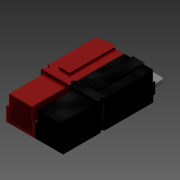
# Autodesk Inventor part: PowerPoles
Saved by Autodesk Inventor 2013 (Build 170138000, 138)
## iProperties
Created: 2012-09-17
Part Number: PowerPoles
Material: Generic
Document SubType Name: Modeling
Designer: Bail
Density: 1 g/cm^3
Author: Bail
Autodesk Inventor part; units mm, degrees
ref_plane "YZ Plane" through (0, 0, 0) normal (1, 0, 0) x (0, 1, 0)
ref_plane "XZ Plane" through (0, 0, 0) normal (0, 1, 0) x (-1, 0, 0)
ref_plane "XY Plane" through (0, 0, 0) normal (0, 0, 1) x (1, 0, 0)
sketch "Sketch1" plane through (0, 0, 0) normal (0, 0, 1) x (1, 0, 0)
  line L0 (-3.937, 3.937) -> (3.937, 3.937)
  line L1 (3.937, 3.937) -> (3.937, -3.937)
  line L2 (3.937, -3.937) -> (-3.937, -3.937)
  line L3 (-3.937, -3.937) -> (-3.937, 3.937)
  point P0 (0, 0)
  dimension "d0" = 7.874
  dimension "d2" = 7.874
  dimension "d3" = 3.937
  dimension "d4" = 3.937
  constraints: 8 end point, 2 parallel, 1 horizontal, 1 perpendicular
  measures "d0" distance of L0.start L0.end
  measures "d2" distance of L0.end L1.end
  measures "d3" distance from line of point (0, 0) L3
  measures "d4" distance from line of point (0, 0) L0
extrude "Extrusion1" add sketch "Sketch1" along normal blind 24.638
sketch "Sketch2" plane through (-3.937, 3.937, 0) normal (0, 1, 0) x (1, 0, 0)
  line L0 (0, 0) -> (7.874, 0) projected
  line L1 (0, 0) -> (0, -24.638) projected
  line L2 (7.874, 0) -> (7.874, -24.638) projected
  line L3 (2.3495, 0) -> (5.5245, 0)
  line L4 (5.5245, 0) -> (5.5245, -12.7)
  line L5 (5.5245, -12.7) -> (2.3495, -12.7)
  line L6 (2.3495, -12.7) -> (2.3495, 0)
  point P0 (3.937, 0)
  dimension "d7" = 3.175
  dimension "d9" = 2.3495
  dimension "d10" = 7.874
  dimension "d11" = 12.7
  constraints: 8 end point, 2 parallel, 1 horizontal, 1 perpendicular, 1 point on line
  measures "d7" distance of L4.end L5.end
  measures "d9" distance between parallel lines of L1 L6
  measures "d10" distance between parallel lines of L2 L1
  measures "d11" distance between parallel lines of L0 L5
extrude "Extrusion2" add sketch "Sketch2" along normal blind 0.508
sketch "Sketch3" plane through (0, 0, 0) normal (0, 0, -1) x (-1, 0, 0)
  line L0 (1.5875, 3.937) -> (1.5875, 4.445) projected
  line L1 (-1.5875, 3.937) -> (-1.5875, 4.445) projected
  line L2 (-1.5875, 3.937) -> (-3.937, 3.937) projected
  line L3 (-1.5875, 3.937) -> (-1.4933, 3.937)
  line L4 (-1.4933, 3.937) -> (1.5875, 3.937)
  line L5 (-1.5875, 4.445) -> (-1.0795, 3.937)
  line L6 (-1.5875, 4.445) -> (-0.8691, 4.445) construction
  line L7 (1.5875, 4.445) -> (1.0795, 3.937)
  line L8 (1.5875, 4.445) -> (2.3059, 4.445) construction
  line L9 (-1.5875, 4.445) -> (-1.5875, 3.937)
  line L10 (1.5875, 4.445) -> (1.5875, 3.937)
  point P0 (0, 0)
  dimension "d14" = 45
  dimension "d15" = 135
  constraints: 16 end point, 3 point on line, 2 collinear, 2 equal length, 2 horizontal, 1 perpendicular
  measures "d14" angle of L5 L6
  measures "d15" angle of L7 L8
extrude "Extrusion3" cut sketch "Sketch3" against normal blind 12.7
sketch "Sketch4" plane through (3.937, -3.937, 0) normal (1, 0, 0) x (0, 0, -1)
  line L0 (-24.638, 7.874) -> (-15.113, 7.874)
  line L1 (-15.113, 7.874) -> (-15.113, 3.937)
  line L2 (-15.113, 3.937) -> (-24.638, 3.937)
  line L3 (-24.638, 3.937) -> (-24.638, 7.874)
  point P0 (0, 3.937)
  dimension "d18" = 9.525
  dimension "d19" = 3.937
  constraints: 8 end point, 2 parallel, 1 horizontal, 1 perpendicular
  measures "d18" distance of L1.end L2.end
  measures "d19" distance of L0.end L1.end
extrude "Extrusion4" cut sketch "Sketch4" against normal blind 12.7
sketch "Sketch5" plane through (0, 0, 0) normal (0, 0, -1) x (-1, 0, 0)
  line L0 (-1.0795, 3.937) -> (-3.937, 3.937) projected
  line L1 (-3.937, 3.937) -> (-3.937, -3.937) projected
  line L2 (-3.937, -3.937) -> (3.937, -3.937) projected
  line L3 (3.937, -3.937) -> (3.937, 3.937) projected
  line L4 (-3.175, 3.175) -> (3.175, 3.175)
  line L5 (3.175, 3.175) -> (3.175, -3.175)
  line L6 (3.175, -3.175) -> (-3.175, -3.175)
  line L7 (-3.175, -3.175) -> (-3.175, 3.175)
  point P0 (0, 0)
  dimension "d22" = 0.762
  dimension "d23" = 0.762
  dimension "d24" = 0.762
  dimension "d25" = 0.762
  constraints: 8 end point, 2 parallel, 1 horizontal, 1 perpendicular
  measures "d22" distance between parallel lines of L3 L5
  measures "d23" distance between parallel lines of L6 L2
  measures "d24" distance between parallel lines of L1 L7
  measures "d25" distance between parallel lines of L0 L4
extrude "Extrusion5" cut sketch "Sketch5" against normal blind 14.605
sketch "Sketch6" plane through (0, 0, 24.638) normal (0, 0, 1) x (1, 0, 0)
  line L0 (3.937, 0) -> (-3.937, 0) projected
  line L1 (-3.937, 0) -> (-3.937, -3.937) projected
  line L2 (-3.937, -3.937) -> (3.937, -3.937) projected
  line L3 (3.937, -3.937) -> (3.937, 0) projected
  line L4 (-3.175, 0) -> (3.175, 0)
  line L5 (3.175, 0) -> (3.175, -3.175)
  line L6 (3.175, -3.175) -> (-3.175, -3.175)
  line L7 (-3.175, -3.175) -> (-3.175, 0)
  point P0 (0, 0)
  dimension "d28" = 0.762
  dimension "d29" = 0.762
  dimension "d30" = 0.762
  constraints: 8 end point, 2 parallel, 1 horizontal, 1 perpendicular, 1 point on line
  measures "d28" distance between parallel lines of L1 L7
  measures "d29" distance between parallel lines of L5 L3
  measures "d30" distance between parallel lines of L2 L6
extrude "Extrusion6" cut sketch "Sketch6" against normal blind 14.605 contours L5 L6 L7 L0
sketch "Sketch7" plane through (3.937, 0, 15.113) normal (0, 0, 1) x (1, 0, 0)
  line L0 (0, 3.937) -> (0, 0) projected
  line L1 (-7.874, 3.937) -> (0, 3.937) projected
  line L2 (-7.112, 0) -> (-0.762, 0)
  line L3 (-0.762, 0) -> (-0.762, 3.175)
  line L4 (-0.762, 3.175) -> (-7.112, 3.175)
  line L5 (-7.112, 3.175) -> (-7.112, 0)
  line L6 (-6.858, 0) -> (-1.016, 0)
  line L7 (-1.016, 0) -> (-1.016, 2.9163)
  line L8 (-1.016, 2.9163) -> (-6.858, 2.9163)
  line L9 (-6.858, 2.9163) -> (-6.858, 0)
  line L10 (-7.112, 3.175) -> (-7.112, 0) projected
  point P0 (-3.937, 0)
  dimension "d33" = 0.762
  dimension "d34" = 0.762
  dimension "d35" = 0.254
  dimension "d36" = 0.2587
  dimension "d37" = 0.254
  constraints: 16 end point, 4 parallel, 2 horizontal, 2 perpendicular, 1 point on line
  measures "d33" distance between parallel lines of L1 L4
  measures "d34" distance between parallel lines of L0 L3
  measures "d35" distance between parallel lines of L9 L10
  measures "d36" distance between parallel lines of L4 L8
  measures "d37" distance between parallel lines of L3 L7
extrude "Extrusion7" add sketch "Sketch7" along normal blind 9.525 contours L5 L4 L3 L2 L7 L8 L9
chamfer "Chamfer1" distance 0.127 angle 45 6 edges at (3.937, 1.9685, 15.113) (3.937, 3.937, 7.5565) (3.937, 0, 0) (3.937, 0, 19.8755) (3.937, -1.9685, 24.638) (3.937, -3.937, 12.319)
sketch "Sketch8" plane through (3.937, -3.81, 0.127) normal (1, 0, 0) x (0, 0, -1)
  line L0 (-24.384, 3.683) -> (-14.859, 3.683) projected
  line L1 (-24.384, 0) -> (-24.384, 3.683) projected
  line L2 (0, 0) -> (-24.384, 0) projected
  line L3 (0, 7.62) -> (0, 0) projected
  line L4 (-14.859, 7.62) -> (0, 7.62) projected
  line L5 (-14.859, 3.683) -> (-14.859, 7.62) projected
  line L6 (0.127, -0.127) -> (0.127, 7.747) projected
  line L7 (0.127, 7.747) -> (-14.986, 7.747) projected
  line L8 (0.127, 7.747) -> (-24.511, 7.747)
  line L9 (-24.511, 7.747) -> (-24.511, -0.127)
  line L10 (-24.511, -0.127) -> (0.127, -0.127)
  line L11 (0.127, -0.127) -> (0.127, 7.747)
  line L12 (-24.511, -0.127) -> (0.127, -0.127) projected
  line L13 (-24.511, 3.81) -> (-24.511, -0.127) projected
  point P0 (0.127, 3.81)
  dimension "d43" = 90
  dimension "d44" = 90
  dimension "d45" = 0
  dimension "d46" = 0
  constraints: 8 end point, 2 parallel, 1 horizontal, 1 perpendicular
  measures "d43" angle of L6 L7
  measures "d44" angle of L12 L13
  measures "d45" distance between parallel lines of L12 L10
  measures "d46" distance between parallel lines of L13 L9
extrude "Extrusion8" add sketch "Sketch8" along normal blind 7.874 contours L0 L5 L4 L3 L2 L1 | L10 L9 L8 L7 L6
sketch "Sketch9" plane through (3.937, -3.937, 0) normal (0, 0, -1) x (-1, 0, 0)
  line L0 (0, 0) -> (0, 7.874) projected
  line L1 (0, 7.874) -> (-7.874, 7.874) projected
  line L2 (-7.874, 0) -> (-7.874, 7.874) projected
  line L3 (-5.5245, 7.874) -> (-2.3495, 7.874)
  line L4 (-2.3495, 7.874) -> (-2.3495, 8.382)
  line L5 (-2.3495, 8.382) -> (-5.5245, 8.382)
  line L6 (-5.5245, 8.382) -> (-5.5245, 7.874)
  line L7 (-5.5245, 8.382) -> (-5.0165, 7.874)
  line L8 (-5.5245, 8.382) -> (-4.8061, 8.382) construction
  line L9 (-2.3495, 8.382) -> (-2.8575, 7.874)
  line L10 (-2.3495, 8.382) -> (-1.6311, 8.382) construction
  point P0 (3.937, 3.937)
  dimension "d49" = 0.508
  dimension "d50" = 3.175
  dimension "d51" = 2.3495
  dimension "d52" = 7.874
  dimension "d53" = 45
  dimension "d54" = 135
  constraints: 16 end point, 3 horizontal, 3 point on line, 2 equal length, 2 parallel, 1 perpendicular
  measures "d49" distance between parallel lines of L1 L5
  measures "d50" distance between parallel lines of L4 L6
  measures "d51" distance between parallel lines of L2 L6
  measures "d52" distance between parallel lines of L0 L2
  measures "d53" angle of L7 L8
  measures "d54" angle of L9 L10
extrude "Extrusion9" add sketch "Sketch9" against normal blind 12.7 contours L1 L7 L5 L9
sketch "Sketch11" plane through (3.937, -3.937, 0) normal (0, 0, -1) x (-1, 0, 0)
  line L0 (0, 0) -> (0, 7.874) projected
  line L1 (-5.0165, 7.874) -> (-7.874, 7.874) projected
  line L2 (-7.874, 0) -> (-7.874, 7.874) projected
  line L3 (0, 0) -> (-7.874, 0) projected
  line L4 (-7.112, 0.762) -> (-0.762, 0.762)
  line L5 (-0.762, 0.762) -> (-0.762, 7.112)
  line L6 (-0.762, 7.112) -> (-7.112, 7.112)
  line L7 (-7.112, 7.112) -> (-7.112, 0.762)
  point P0 (3.937, 3.937)
  dimension "d57" = 0.762
  dimension "d58" = 0.762
  dimension "d59" = 0.762
  dimension "d60" = 0.762
  constraints: 8 end point, 2 parallel, 1 horizontal, 1 perpendicular
  measures "d57" distance between parallel lines of L2 L7
  measures "d58" distance between parallel lines of L4 L3
  measures "d59" distance between parallel lines of L5 L0
  measures "d60" distance between parallel lines of L6 L1
extrude "Extrusion10" cut sketch "Sketch11" against normal blind 14.605
sketch "Sketch12" plane through (3.937, -3.937, 24.638) normal (0, 0, 1) x (1, 0, 0)
  line L0 (0, 7.874) -> (0, 0) projected
  line L1 (0, 0) -> (7.874, 0) projected
  line L2 (7.874, 7.874) -> (7.874, 0) projected
  line L3 (0, 7.874) -> (7.874, 7.874) projected
  line L4 (0.762, 7.112) -> (7.112, 7.112)
  line L5 (7.112, 7.112) -> (7.112, 3.937)
  line L6 (7.112, 3.937) -> (0.762, 3.937)
  line L7 (0.762, 3.937) -> (0.762, 7.112)
  line L8 (-7.874, 0) -> (-0.127, 0) projected
  line L9 (-1.016, 3.937) -> (-6.858, 3.937) projected
  line L10 (-0.762, 3.937) -> (-0.762, 7.112) projected
  line L11 (-7.112, 7.112) -> (-7.112, 3.937) projected
  line L12 (-0.762, 7.112) -> (-7.112, 7.112) projected
  line L13 (1.016, 3.937) -> (6.858, 3.937)
  line L14 (6.858, 3.937) -> (6.858, 6.858)
  line L15 (6.858, 6.858) -> (1.016, 6.858)
  line L16 (1.016, 6.858) -> (1.016, 3.937)
  line L17 (-6.858, 3.937) -> (-6.858, 6.8533) projected
  line L18 (0, 3.937) -> (7.874, 3.937)
  line L19 (0, 7.874) -> (0, 3.937)
  line L20 (0, 7.874) -> (7.874, 7.874)
  line L21 (7.874, 7.874) -> (7.874, 3.937)
  line L22 (0.762, 3.937) -> (7.112, 3.937)
  line L23 (7.112, 3.937) -> (7.112, 0.762)
  line L24 (7.112, 0.762) -> (0.762, 0.762)
  line L25 (0.762, 0.762) -> (0.762, 3.937)
  point P0 (-3.937, 3.937)
  dimension "d63" = 3.937
  dimension "d64" = 3.937
  dimension "d65" = 6.35
  dimension "d66" = 6.35
  dimension "d67" = 7.874
  dimension "d68" = 0.762
  dimension "d69" = 3.175
  dimension "d70" = 3.175
  dimension "d71" = 0.254
  dimension "d72" = 0.254
  dimension "d73" = 0.254
  dimension "d74" = 0.254
  dimension "d77" = 0.762
  dimension "d78" = 0.762
  constraints: 32 end point, 7 equal length, 5 perpendicular, 3 horizontal, 2 midpoint, 1 point on line
  measures "d63" distance between parallel lines of L8 L9
  measures "d64" distance between parallel lines of L1 L6
  measures "d65" distance between parallel lines of L10 L11
  measures "d66" distance of L4.start L4.end
  measures "d67" distance of L0.start L2.start
  measures "d68" distance between parallel lines of L7 L0
  measures "d69" distance between parallel lines of L9 L12
  measures "d70" distance between parallel lines of L6 L4
  measures "d71" distance between parallel lines of L11 L17
  measures "d72" distance between parallel lines of L7 L16
  measures "d73" distance between parallel lines of L4 L15
  measures "d74" distance between parallel lines of L5 L14
  measures "d77" distance between parallel lines of L24 L1
  measures "d78" distance between parallel lines of L2 L23
extrude "Extrusion11" cut sketch "Sketch12" against normal blind 9.525 contours L3 L2 L18 L5 L4 L7 L0 | L6 L23 L24 L25 | L16 L15 L14 L6
sketch "Sketch13" plane through (3.937, -3.937, 15.113) normal (0, 0, 1) x (1, 0, 0)
  line L0 (0.762, 3.937) -> (7.112, 3.937)
  line L1 (7.112, 3.937) -> (7.112, 0.762)
  line L2 (7.112, 0.762) -> (0.762, 0.762)
  line L3 (0.762, 0.762) -> (0.762, 3.937)
  point P0 (-3.937, 3.937)
  constraints: 8 end point, 2 parallel, 1 horizontal, 1 perpendicular
extrude "Extrusion12" cut sketch "Sketch13" against normal blind 9.525
chamfer "Chamfer2" distance 0.127 angle 45 6 edges at (3.937, 3.937, 7.5565) (3.937, 0, 19.8755) (3.81, 0, 19.8755) (11.811, 0, 19.8755) (11.811, -3.937, 12.319) (11.811, 3.937, 7.5565)
sketch "Sketch14" plane through (0, 0, 0) normal (0, 0, -1) x (-1, 0, 0)
  line L0 (-3.81, -3.937) -> (3.937, -3.937) projected
  line L1 (3.937, -3.937) -> (3.937, 3.937) projected
  line L2 (3.937, 3.937) -> (1.0795, 3.937) projected
  line L3 (-1.5875, 4.445) -> (-1.0795, 3.937) projected
  line L4 (3.937, 1.5875) -> (3.429, 1.5875)
  line L5 (3.429, 1.5875) -> (3.429, -1.5875)
  line L6 (3.429, -1.5875) -> (3.937, -1.5875)
  line L7 (3.937, -1.5875) -> (3.937, 1.5875)
  line L8 (3.429, 1.5875) -> (3.937, 1.0795)
  line L9 (3.429, -1.5875) -> (3.937, -1.0795)
  point P0 (0, 0)
  dimension "d67" = 7.874
  dimension "d84" = 0.508
  dimension "d85" = 3.175
  dimension "d86" = 2.3495
  dimension "d87" = 7.874
  constraints: 12 end point, 3 parallel, 3 point on line, 2 perpendicular, 1 horizontal
  measures "d84" distance of L6.end L5.end
  measures "d85" distance of L5.end L4.end
  measures "d86" distance between parallel lines of L4 L2
  measures "d87" distance between parallel lines of L0 L2
extrude "Extrusion13" cut sketch "Sketch14" against normal blind 12.7 contours L9 L5 L8 L1
sketch "Sketch15" plane through (9.4615, 4.445, 0) normal (0, 0, -1) x (-1, 0, 0)
  line L0 (-2.3495, -8.255) -> (-2.3495, -0.635) projected
  line L1 (5.5245, -8.382) -> (-2.2225, -8.382) projected
  line L2 (0, 0) -> (0.508, -0.508) projected
  line L3 (0.508, -0.508) -> (-2.2225, -0.508) projected
  line L4 (-2.3495, -2.8575) -> (-2.8575, -2.8575)
  line L5 (-2.8575, -2.8575) -> (-2.8575, -6.0325)
  line L6 (-2.8575, -6.0325) -> (-2.3495, -6.0325)
  line L7 (-2.3495, -6.0325) -> (-2.3495, -2.8575)
  line L8 (-2.8575, -2.8575) -> (-2.3495, -3.3655)
  line L9 (-2.8575, -6.0325) -> (-2.3495, -5.5245)
  point P0 (9.4615, -4.445)
  dimension "d90" = 0.508
  dimension "d91" = 3.175
  dimension "d92" = 7.874
  dimension "d93" = 2.3495
  constraints: 12 end point, 3 parallel, 3 point on line, 2 perpendicular, 1 horizontal
  measures "d90" distance between parallel lines of L0 L5
  measures "d91" distance between parallel lines of L4 L6
  measures "d92" distance between parallel lines of L1 L3
  measures "d93" distance between parallel lines of L1 L6
extrude "Extrusion14" add sketch "Sketch15" against normal blind 12.7 contours L9 L5 L8 L0
sketch "Sketch16" plane through (9.4615, 4.445, 0) normal (0, 0, -1) x (-1, 0, 0)
  line L0 (-2.3495, -8.255) -> (-2.3495, -5.5245) projected
  line L1 (5.5245, -8.382) -> (-2.2225, -8.382) projected
  line L2 (5.5245, -8.382) -> (5.5245, -0.635) projected
  line L3 (0, 0) -> (0.508, -0.508) projected
  line L4 (0, -8.382) -> (3.175, -8.382)
  line L5 (3.175, -8.382) -> (3.175, -7.874)
  line L6 (3.175, -7.874) -> (0, -7.874)
  line L7 (0, -7.874) -> (0, -8.382)
  line L8 (0, -7.874) -> (0.508, -8.382)
  line L9 (3.175, -7.874) -> (2.667, -8.382)
  point P0 (9.4615, -4.445)
  dimension "d96" = 3.175
  dimension "d98" = 7.874
  dimension "d99" = 2.3495
  dimension "d100" = 0.508
  constraints: 12 end point, 3 parallel, 3 point on line, 2 perpendicular, 1 horizontal
  measures "d96" distance of L5.end L6.end
  measures "d98" distance between parallel lines of L2 L0
  measures "d99" distance between parallel lines of L0 L7
  measures "d100" distance between parallel lines of L4 L6
extrude "Extrusion15" cut sketch "Sketch16" against normal blind 12.7 contours L1 L8 L6 L9
sketch "Sketch17" plane through (0, 0, 0) normal (0, 0, -1) x (-1, 0, 0)
  line L0 (-3.81, -3.937) -> (3.937, -3.937) projected
  line L1 (3.937, -3.937) -> (3.937, -1.0795) projected
  line L2 (3.937, -1.0795) -> (3.429, -1.5875) projected
  line L3 (-1.5875, -3.937) -> (1.5875, -3.937)
  line L4 (1.5875, -3.937) -> (1.5875, -3.429)
  line L5 (1.5875, -3.429) -> (-1.5875, -3.429)
  line L6 (-1.5875, -3.429) -> (-1.5875, -3.937)
  line L7 (-3.937, -3.937) -> (-3.937, 3.81) projected
  line L8 (-1.5875, -3.429) -> (-1.0795, -3.937)
  line L9 (1.5875, -3.429) -> (1.0795, -3.937)
  point P0 (0, 0)
  dimension "d103" = 3.175
  dimension "d104" = 7.874
  dimension "d105" = 0.508
  dimension "d106" = 2.3495
  constraints: 12 end point, 3 perpendicular, 3 point on line, 2 parallel, 1 horizontal
  measures "d103" distance of L5.end L4.end
  measures "d104" distance between parallel lines of L1 L7
  measures "d105" distance of L3.end L4.end
  measures "d106" distance between parallel lines of L1 L4
extrude "Extrusion16" cut sketch "Sketch17" against normal blind 12.7 contours L8 L5 L9 L0
chamfer "Chamfer3" distance 0.127 angle 45 15 edges at (3.81, 3.937, 7.5565) (-3.937, 3.937, 7.5565) (-3.937, 0, 19.8755) (3.937, -3.937, 12.319) (3.81, -3.937, 12.319) (3.937, -0.0634, 0) (3.81, 0, 0) (5.4292, 3.937, 0) (2.4447, 3.937, 0) (-2.5083, 3.937, 0) (11.811, 2.4448, 0) (4.699, 3.175, 19.8755) (3.175, 3.175, 19.8755) (-3.175, 3.175, 19.8755) (11.049, 3.175, 19.8755)
sketch "Sketch18" plane through (-1.0795, 3.937, 12.7) normal (0, 1, 0) x (1, 0, 0)
  line L0 (-2.7305, -2.413) -> (-2.7305, 12.573) projected
  line L1 (-2.8575, 12.7) -> (-2.8575, -2.413) projected
  line L2 (5.0165, -2.286) -> (5.0165, 12.573) projected
  line L3 (12.8905, -2.413) -> (12.8905, 12.573) projected
  circle A0 centre (5.0165, -1.143) radius 0.635
  line L4 (4.7625, 12.7) -> (2.032, 12.7) projected
  circle A1 centre (12.8905, -1.143) radius 0.635
  circle A2 centre (-2.7305, -1.143) radius 0.635
  point P0 (1.0795, 12.7)
  dimension "d112" = 7.874
  dimension "d113" = 7.874
  dimension "d114" = 1.27
  dimension "d115" = 13.843
  dimension "d116" = 1.27
  dimension "d117" = 13.843
  dimension "d118" = 1.27
  constraints: 3 centre point, 3 point on line
  measures "d112" distance between parallel lines of L1 L2
  measures "d113" distance between parallel lines of L2 L3
  measures "d114" diameter of A0
  measures "d115" distance from line of L4 A0.centre
  measures "d116" diameter of A1
  measures "d117" distance from line of L4 A1.centre
  measures "d118" diameter of A2
extrude "Extrusion17" cut sketch "Sketch18" against normal through all
sketch "Sketch19" plane through (0, 0, 0) normal (0, 0, -1) x (-1, 0, 0)
  line L0 (1.0795, -3.937) -> (3.937, -3.937) projected
  line L1 (-1.905, -1.651) -> (1.905, -1.651)
  line L2 (1.905, -1.651) -> (1.905, -2.667)
  line L3 (1.905, -2.667) -> (-1.905, -2.667)
  line L4 (-1.905, -2.667) -> (-1.905, -1.651)
  line L5 (-9.779, -1.651) -> (-5.969, -1.651)
  line L6 (-5.969, -1.651) -> (-5.969, -2.667)
  line L7 (-5.969, -2.667) -> (-9.779, -2.667)
  line L8 (-9.779, -2.667) -> (-9.779, -1.651)
  line L9 (-3.937, 3.81) -> (-3.937, -3.81) projected
  line L10 (-11.811, 3.81) -> (-11.811, 1.0795) projected
  point P0 (0, 0)
  point P1 (-8.9535, -3.937)
  dimension "d121" = 3.81
  dimension "d123" = 3.81
  dimension "d124" = 7.874
  dimension "d125" = 2.032
  dimension "d126" = 2.032
  dimension "d127" = 1.016
  dimension "d128" = 1.016
  dimension "d129" = 1.27
  dimension "d130" = 1.27
  constraints: 16 end point, 4 parallel, 2 horizontal, 2 perpendicular
  measures "d121" distance of L1.start L1.end
  measures "d123" distance of L5.start L5.end
  measures "d124" distance between parallel lines of L9 L10
  measures "d125" distance between parallel lines of L10 L8
  measures "d126" distance between parallel lines of L4 L9
  measures "d127" distance between parallel lines of L3 L1
  measures "d128" distance between parallel lines of L7 L5
  measures "d129" distance between parallel lines of L0 L3
  measures "d130" distance from line of point (-8.954, -3.937) L7
extrude "Extrusion18" add sketch "Sketch19" along normal blind 5.08
chamfer "Chamfer4" distance 0.508 angle 45 4 edges at (9.779, -2.159, -5.08) (5.969, -2.159, -5.08) (1.905, -2.159, -5.08) (-1.905, -2.159, -5.08)
equation "\"d3\" = 0.5 * d0"
equation "\"d4\" = 0.5 * d2"
equation "\"d9\" = 0.5 * d10 - 0.5 * d7"
equation "\"d51\" = 0.5 * d52 - 0.5 * d50"
equation "\"d64\" = d63"
equation "\"d66\" = d65"
equation "\"d68\" = 0.5 * d67 - 0.5 * d66"
equation "\"d70\" = d69"
equation "\"d72\" = d71"
equation "\"d73\" = d71"
equation "\"d74\" = d71"
equation "\"d86\" = 0.5 * d87 - 0.5 * d85"
equation "\"d93\" = 0.5 * d92 - 0.5 * d91"
equation "\"d99\" = 0.5 * d98 - 0.5 * d96"
equation "\"d106\" = 0.5 * d104 - 0.5 * d103"
equation "\"d116\" = d114"
equation "\"d117\" = d115"
equation "\"d125\" = 0.5 * d124 - 0.5 * d123"
equation "\"d126\" = d125"
body "Solid1"
